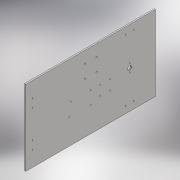
# Autodesk Inventor part: 290mm板
Saved by Autodesk Inventor 2017 (Build 210142000, 142)
## iProperties
Part Number: 290mm板
Material: 常规
Document SubType Name: 钣金
Designer: PANDA
Density: 1 g/cm^3
Sheet Metal Rule: 默认_mm
Appearance: 默认
Author: PANDA
Autodesk Inventor part; units mm, degrees
ref_plane "YZ Plane" through (0, 0, 0) normal (1, 0, 0) x (0, 1, 0)
ref_plane "XZ Plane" through (0, 0, 0) normal (0, 1, 0) x (-1, 0, 0)
ref_plane "XY Plane" through (0, 0, 0) normal (0, 0, 1) x (1, 0, 0)
sketch "草图1" plane through (0, 0, 0) normal (1, 0, 0) x (0, 1, 0)
  line L0 (250, 140) -> (-250, 140)
  line L1 (-250, 140) -> (-250, -150)
  line L2 (-250, -150) -> (250, -150)
  line L3 (250, -150) -> (250, 140)
  point P0 (0, 0)
  dimension "d0" = 500
  dimension "d1" = 290
  constraints: 8 end point, 2 parallel, 1 horizontal, 1 perpendicular
  measures "d0" distance of L2.end L1.end
  measures "d1" distance of L1.end L0.end
extrude "拉伸1" add sketch "草图1" along normal blind 5
sketch "草图2" plane through (5, 0, 0) normal (1, 0, 0) x (0, 0, -1)
  circle A0 centre (85.5, -224) radius 1.8
  point P0 (0, 0)
  dimension "d4" = 3.6
  constraints: 1 centre point
  measures "d4" diameter of A0
extrude "拉伸2" cut sketch "草图2" against normal through all
sketch "草图3" plane through (5, 0, 0) normal (1, 0, 0) x (0, 0, -1)
  circle A0 centre (-85.5, -224) radius 1.8
  point P0 (0, 0)
  dimension "d7" = 3.6
  constraints: 1 centre point
  measures "d7" diameter of A0
extrude "拉伸3" cut sketch "草图3" against normal through all
sketch "草图4" plane through (0, 0, 0) normal (-1, 0, 0) x (0, 0, 1)
  circle A0 centre (54.5, -224) radius 1.8
  point P0 (0, 0)
  dimension "d10" = 3.6
  constraints: 1 centre point
  measures "d10" diameter of A0
extrude "拉伸4" cut sketch "草图4" against normal through all
sketch "草图5" plane through (5, 0, 0) normal (1, 0, 0) x (0, 0, -1)
  circle A0 centre (54.5, -224) radius 1.8
  point P0 (0, 0)
  dimension "d13" = 3.6
  constraints: 1 centre point
  measures "d13" diameter of A0
extrude "拉伸5" cut sketch "草图5" against normal through all
sketch "草图8" plane through (5, 0, 0) normal (1, 0, 0) x (0, 0, -1)
  circle A0 centre (-119, 165.5) radius 1.8
  point P0 (0, 0)
  dimension "d22" = 3.6
  constraints: 1 centre point
  measures "d22" diameter of A0
extrude "拉伸8" cut sketch "草图8" against normal through all
sketch "草图9" plane through (0, 0, 0) normal (-1, 0, 0) x (0, 0, 1)
  circle A0 centre (119, 134.5) radius 1.8
  point P0 (0, 0)
  dimension "d25" = 3.6
  constraints: 1 centre point
  measures "d25" diameter of A0
extrude "拉伸9" cut sketch "草图9" against normal through all
sketch "草图10" plane through (5, 0, 0) normal (1, 0, 0) x (0, 0, -1)
  circle A0 centre (119, 134.5) radius 1.8
  point P0 (0, 0)
  dimension "d28" = 3.6
  constraints: 1 centre point
  measures "d28" diameter of A0
extrude "拉伸10" cut sketch "草图10" against normal through all
sketch "草图11" plane through (5, 0, 0) normal (1, 0, 0) x (0, 0, -1)
  circle A0 centre (119, 165.5) radius 1.8
  point P0 (0, 0)
  dimension "d31" = 3.6
  constraints: 1 centre point
  measures "d31" diameter of A0
extrude "拉伸11" cut sketch "草图11" against normal through all
sketch "草图12" plane through (5, 0, 0) normal (1, 0, 0) x (0, 0, -1)
  line L0 (145, -250) -> (150, -250)
  line L1 (150, -250) -> (150, 250)
  line L2 (150, 250) -> (145, 250)
  line L3 (145, 250) -> (145, -250)
  point P0 (0, 0)
  dimension "d34" = 5
  dimension "d35" = 500
  constraints: 8 end point, 2 parallel, 1 horizontal, 1 perpendicular
  measures "d34" distance of L2.end L1.end
  measures "d35" distance of L1.end L0.end
extrude "拉伸12" cut sketch "草图12" against normal through all
sketch "草图13" plane through (5, 0, 0) normal (1, 0, 0) x (0, 0, -1)
  line L0 (-140, -250) -> (-145, -250)
  line L1 (-145, -250) -> (-145, 250)
  line L2 (-145, 250) -> (-140, 250)
  line L3 (-140, 250) -> (-140, -250)
  point P0 (0, 0)
  dimension "d38" = 5
  dimension "d39" = 500
  constraints: 8 end point, 2 parallel, 1 horizontal, 1 perpendicular
  measures "d38" distance of L1.end L2.end
  measures "d39" distance of L0.end L1.end
extrude "拉伸13" add sketch "草图13" against normal blind 5
sketch "草图14" plane through (5, 0, 0) normal (1, 0, 0) x (0, 0, -1)
  circle A0 centre (0, 0) radius 1.8
  dimension "d42" = 3.6
  constraints: 1 centre point, 1 coincident
  measures "d42" diameter of A0
extrude "拉伸14" cut sketch "草图14" against normal through all
sketch "草图15" plane through (5, 0, 0) normal (1, 0, 0) x (0, 0, -1)
  circle A0 centre (48.4, 0) radius 1.8
  point P0 (0, 0)
  dimension "d45" = 3.6
  constraints: 1 centre point
  measures "d45" diameter of A0
extrude "拉伸15" cut sketch "草图15" against normal through all
sketch "草图16" plane through (5, 0, 0) normal (1, 0, 0) x (0, 0, -1)
  circle A0 centre (0, -74.8) radius 1.8
  point P0 (0, 0)
  dimension "d48" = 3.6
  constraints: 1 centre point
  measures "d48" diameter of A0
extrude "拉伸16" cut sketch "草图16" against normal through all
sketch "草图17" plane through (5, 0, 0) normal (1, 0, 0) x (0, 0, -1)
  circle A0 centre (48.4, -81.8) radius 1.8
  point P0 (0, 0)
  dimension "d51" = 3.6
  constraints: 1 centre point
  measures "d51" diameter of A0
extrude "拉伸17" cut sketch "草图17" against normal through all
sketch "草图18" plane through (5, 0, 0) normal (1, 0, 0) x (0, 0, -1)
  circle A0 centre (0, 37) radius 1.8
  point P0 (0, 0)
  dimension "d54" = 3.6
  constraints: 1 centre point
  measures "d54" diameter of A0
extrude "拉伸18" cut sketch "草图18" against normal through all
sketch "草图19" plane through (5, 0, 0) normal (1, 0, 0) x (0, 0, -1)
  circle A0 centre (37, 74) radius 1.8
  point P0 (0, 0)
  dimension "d57" = 3.6
  constraints: 1 centre point
  measures "d57" diameter of A0
extrude "拉伸19" cut sketch "草图19" against normal through all
sketch "草图20" plane through (5, 0, 0) normal (1, 0, 0) x (0, 0, -1)
  circle A0 centre (0, 74) radius 1.8
  point P0 (0, 0)
  dimension "d60" = 3.6
  constraints: 1 centre point
  measures "d60" diameter of A0
extrude "拉伸20" cut sketch "草图20" against normal through all
sketch "草图21" plane through (5, 0, 0) normal (1, 0, 0) x (0, 0, -1)
  circle A0 centre (37, 37) radius 1.8
  point P0 (0, 0)
  dimension "d63" = 3.6
  constraints: 1 centre point
  measures "d63" diameter of A0
extrude "拉伸21" cut sketch "草图21" against normal through all
sketch "草图22" plane through (5, 0, 0) normal (1, 0, 0) x (0, 0, -1)
  circle A0 centre (-50, -22.5) radius 2.5
  point P0 (0, 0)
  dimension "d66" = 5
  constraints: 1 centre point
  measures "d66" diameter of A0
extrude "拉伸22" cut sketch "草图22" against normal through all
sketch "草图23" plane through (5, 0, 0) normal (1, 0, 0) x (0, 0, -1)
  circle A0 centre (-50, 22.5) radius 2.5
  point P0 (0, 0)
  dimension "d69" = 5
  constraints: 1 centre point
  measures "d69" diameter of A0
extrude "拉伸23" cut sketch "草图23" against normal through all
sketch "草图24" plane through (5, 0, 0) normal (1, 0, 0) x (0, 0, -1)
  circle A0 centre (-100, -22.5) radius 2.5
  point P0 (0, 0)
  dimension "d72" = 5
  constraints: 1 centre point
  measures "d72" diameter of A0
extrude "拉伸24" cut sketch "草图24" against normal through all
sketch "草图25" plane through (5, 0, 0) normal (1, 0, 0) x (0, 0, -1)
  circle A0 centre (-100, 22.5) radius 2.5
  point P0 (0, 0)
  dimension "d75" = 5
  constraints: 1 centre point
  measures "d75" diameter of A0
extrude "拉伸25" cut sketch "草图25" against normal through all
sketch "草图26" plane through (5, 0, 0) normal (1, 0, 0) x (0, 0, -1)
  circle A0 centre (15.5, 150) radius 1.8
  point P0 (0, 0)
  dimension "d78" = 3.6
  constraints: 1 centre point
  measures "d78" diameter of A0
extrude "拉伸26" cut sketch "草图26" against normal through all
sketch "草图27" plane through (5, 0, 0) normal (1, 0, 0) x (0, 0, -1)
  circle A0 centre (-15.5, 150) radius 1.8
  point P0 (0, 0)
  dimension "d81" = 3.6
  constraints: 1 centre point
  measures "d81" diameter of A0
extrude "拉伸27" cut sketch "草图27" against normal through all
sketch "草图28" plane through (5, 0, 0) normal (1, 0, 0) x (0, 0, -1)
  circle A0 centre (0, 150) radius 7.5
  point P0 (0, 0)
  dimension "d84" = 15
  constraints: 1 centre point
  measures "d84" diameter of A0
extrude "拉伸28" cut sketch "草图28" against normal through all
equation "\"折弯半径\" = 厚度"
equation "\"折弯释压宽度\" = 厚度"
equation "\"折弯释压深度\" = 0.5 * 厚度"
equation "\"拐角释压尺寸\" = 4 * 厚度"
equation "\"最小余量\" = 2 * 厚度"
equation "\"过渡半径\" = 折弯半径"
equation "\"Jacobi半径尺寸\" = 折弯半径"
equation "\"间隙大小\" = 厚度"
equation "\"厚度\" = 0.5"
